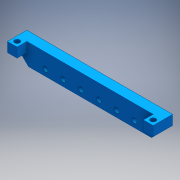
# Autodesk Inventor part: frameBottomRight
Saved by Autodesk Inventor 2016 (Build 200138000, 138)
## iProperties
Created: 2016-05-25
Part Number: frameBottomRight
Material: ABS Plastic
Document SubType Name: Modeling
Designer: Henrik Samuelsson
Density: 1.06 g/cm^3
Appearance: Smooth - White
Author: Henrik Samuelsson
Autodesk Inventor part; units mm, degrees
ref_plane "YZ Plane" through (0, 0, 0) normal (1, 0, 0) x (0, 1, 0)
ref_plane "XZ Plane" through (0, 0, 0) normal (0, 1, 0) x (-1, 0, 0)
ref_plane "XY Plane" through (0, 0, 0) normal (0, 0, 1) x (1, 0, 0)
sketch "Sketch5" plane through (0, 0, 0) normal (0, 1, 0) x (-1, 0, 0)
  line L0 (0, 0) -> (180, 0)
  line L1 (180, 0) -> (180, -12)
  line L2 (0, -12) -> (0, 0)
  line L3 (166, -26) -> (14, -26)
  line L4 (0, -12) -> (14, -26)
  line L5 (180, -12) -> (166, -26)
  circle A0 centre (101, -18) radius 3
  circle A1 centre (79, -18) radius 3
  circle A2 centre (57, -18) radius 3
  circle A3 centre (123, -18) radius 3
  circle A4 centre (145, -18) radius 3
  circle A5 centre (35, -18) radius 3
  dimension "d57" = 6
  dimension "d58" = 79
  dimension "d59" = 180
  dimension "d60" = 12
  dimension "d61" = 14
  dimension "d62" = 14
  dimension "d63" = 14
  dimension "d64" = 14
  dimension "d65" = 152
  dimension "d66" = 8
  dimension "d67" = 6
  dimension "d68" = 6
  dimension "d69" = 6
  dimension "d70" = 6
  dimension "d71" = 8
  dimension "d72" = 8
  dimension "d73" = 8
  dimension "d74" = 8
  dimension "d75" = 22
  dimension "d76" = 22
  dimension "d77" = 22
  dimension "d78" = 22
  dimension "d95" = 6
  dimension "d96" = 0
  dimension "d97" = 22
  constraints: 12 end point, 6 centre point, 1 horizontal, 1 parallel, 1 perpendicular
  measures "d57" diameter of A0
  measures "d58" distance from line of L1 A0.centre
  measures "d59" distance of L0.end L0.start
  measures "d60" distance of L0.start L2.start
  measures "d61" horizontal distance of L2.start L3.end
  measures "d62" horizontal distance of L1.end L3.start
  measures "d63" horizontal distance of L1.end L3.start
  measures "d64" horizontal distance of L3.end L2.start
  measures "d65" distance of L3.start L3.end
  measures "d66" distance from line of L3 A0.centre
  measures "d67" diameter of A1
  measures "d68" diameter of A2
  measures "d69" diameter of A3
  measures "d70" diameter of A4
  measures "d71" distance from line of L3 A2.centre
  measures "d72" distance from line of L3 A1.centre
  measures "d73" distance from line of L3 A3.centre
  measures "d74" distance from line of L3 A4.centre
  measures "d75" distance of A0.centre A1.centre
  measures "d76" distance of A1.centre A2.centre
  measures "d77" distance of A3.centre A0.centre
  measures "d78" distance of A4.centre A3.centre
  measures "d95" diameter of A5
  measures "d96" vertical distance of A2.centre A5.centre
  measures "d97" distance of A2.centre A5.centre
extrude "Extrusion7" add sketch "Sketch5" along normal blind 12
sketch "Sketch8" plane through (0, 0, 0) normal (0, -1, 0) x (1, 0, 0)
  line L0 (0, 0) -> (0, -12) projected
  line L1 (0, 0) -> (-12, 0)
  line L2 (-12, 0) -> (-12, -12)
  line L3 (-12, -12) -> (0, -12)
  line L4 (0, -12) -> (0, 0)
  line L5 (-180, -12) -> (-180, 0) projected
  line L6 (-180, 0) -> (-168, 0)
  line L7 (-168, 0) -> (-168, -12)
  line L8 (-168, -12) -> (-180, -12)
  line L9 (-180, -12) -> (-180, 0)
  dimension "d100" = 12
  dimension "d101" = 12
  dimension "d102" = 12
  dimension "d103" = 12
  constraints: 16 end point, 4 parallel, 2 horizontal, 2 perpendicular
  measures "d100" distance of L3.end L2.end
  measures "d101" distance of L2.end L1.end
  measures "d102" distance of L7.end L8.end
  measures "d103" distance of L6.end L7.end
extrude "Extrusion8" add sketch "Sketch8" along normal blind 12
sketch "Sketch11" plane through (0, 12, 0) normal (0, 1, 0) x (1, 0, 0)
  circle A0 centre (-35, 18) radius 3 projected
  line L0 (-38.0022, 12.8) -> (-41.0044, 18)
  line L1 (-41.0044, 18) -> (-38.0022, 23.2)
  line L2 (-38.0022, 23.2) -> (-31.9978, 23.2)
  line L3 (-31.9978, 23.2) -> (-28.9956, 18)
  line L4 (-28.9956, 18) -> (-31.9978, 12.8)
  line L5 (-31.9978, 12.8) -> (-38.0022, 12.8)
  circle A1 centre (-57, 18) radius 3 projected
  line L6 (-60.0022, 12.8) -> (-63.0044, 18)
  line L7 (-63.0044, 18) -> (-60.0022, 23.2)
  line L8 (-60.0022, 23.2) -> (-53.9978, 23.2)
  line L9 (-53.9978, 23.2) -> (-50.9956, 18)
  line L10 (-50.9956, 18) -> (-53.9978, 12.8)
  line L11 (-53.9978, 12.8) -> (-60.0022, 12.8)
  line L12 (-75.9978, 12.8) -> (-82.0022, 12.8)
  line L13 (-82.0022, 12.8) -> (-85.0044, 18)
  line L14 (-85.0044, 18) -> (-82.0022, 23.2)
  line L15 (-82.0022, 23.2) -> (-75.9978, 23.2)
  line L16 (-75.9978, 23.2) -> (-72.9956, 18)
  line L17 (-72.9956, 18) -> (-75.9978, 12.8)
  circle A2 centre (-101, 18) radius 3 projected
  line L18 (-104.0022, 12.8) -> (-107.0044, 18)
  line L19 (-107.0044, 18) -> (-104.0022, 23.2)
  line L20 (-104.0022, 23.2) -> (-97.9978, 23.2)
  line L21 (-97.9978, 23.2) -> (-94.9956, 18)
  line L22 (-94.9956, 18) -> (-97.9978, 12.8)
  line L23 (-97.9978, 12.8) -> (-104.0022, 12.8)
  circle A3 centre (-123, 18) radius 3 projected
  line L24 (-119.9978, 12.8) -> (-126.0022, 12.8)
  line L25 (-126.0022, 12.8) -> (-129.0044, 18)
  line L26 (-129.0044, 18) -> (-126.0022, 23.2)
  line L27 (-126.0022, 23.2) -> (-119.9978, 23.2)
  line L28 (-119.9978, 23.2) -> (-116.9956, 18)
  line L29 (-116.9956, 18) -> (-119.9978, 12.8)
  circle A4 centre (-145, 18) radius 3 projected
  line L30 (-148.0022, 12.8) -> (-151.0044, 18)
  line L31 (-151.0044, 18) -> (-148.0022, 23.2)
  line L32 (-148.0022, 23.2) -> (-141.9978, 23.2)
  line L33 (-141.9978, 23.2) -> (-138.9956, 18)
  line L34 (-138.9956, 18) -> (-141.9978, 12.8)
  line L35 (-141.9978, 12.8) -> (-148.0022, 12.8)
  point P0 (0, 0)
  point P1 (-79, 18)
  dimension "d123" = 5.2
  dimension "d125" = 5.2
  dimension "d126" = 5.2
  dimension "d127" = 5.2
  dimension "d128" = 5.2
  dimension "d129" = 22
  constraints: 72 end point, 6 horizontal, 5 coincident, 2 point on line, 78 other
  measures "d123" distance from line of L5 point (-35, 18)
  measures "d125" distance from line of L11 point (-57, 18)
  measures "d126" distance from line of L12 point (-79, 18)
  measures "d127" distance from line of L24 point (-123, 18)
  measures "d128" distance from line of L35 point (-145, 18)
  measures "d129" distance of point (-79, 18) A1.centre
extrude "Extrusion11" cut sketch "Sketch11" against normal blind 5
hole "Hole3" at (-6, -6, 0) direction (0, 0, -1) diameter 6.4 depth 12 tip angle 118
hole "Hole4" at (-174, -6, 0) direction (0, 0, -1) diameter 6.4 depth 12 tip angle 118
body "Solid2"
